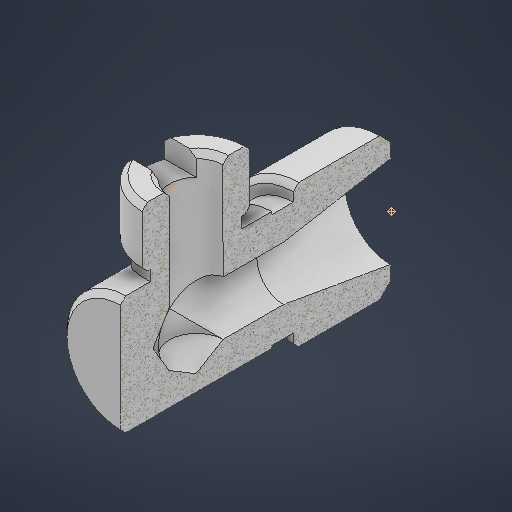
# Autodesk Inventor part: b5
Saved by Autodesk Inventor 2025.4 (Build 294407000, 407)
## iProperties
Created: 2026-05-15
Part Number: b5
Material: Generic
Document SubType Name: Modeling
Designer: VuQuan
Density: 1 g/cm^3
Appearance: Default
Author: VuQuan
Autodesk Inventor part; units mm, degrees
ref_plane "YZ Plane" through (0, 0, 0) normal (1, 0, 0) x (0, 1, 0)
ref_plane "XY Plane" through (0, 0, 0) normal (0, 0, 1) x (1, 0, 0)
sketch "Sketch1" plane through (0, 0, 0) normal (0, 0, 1) x (1, 0, 0)
  circle A0 centre (0, 0) radius 6.58
  circle A1 centre (0, 0) radius 5.5
  circle A2 centre (0, 0) radius 5.25
  dimension "d0" = 13.16
  dimension "d1" = 11
  dimension "d2" = 10.5
  constraints: 3 centre point, 3 coincident
  measures "d0" diameter of A0
  measures "d1" diameter of A1
  measures "d2" diameter of A2
extrude "Extrusion1" add sketch "Sketch1" along normal blind 9 contours A0 | A1 | A2
extrude "Extrusion2" add sketch "Sketch1" along normal blind 2 from surface at 9 contours A2
extrude "Extrusion3" add sketch "Sketch1" along normal blind 14 from surface at 11 contours A1 | A2
sketch "Sketch7" plane through (0, 0, 0) normal (1, 0, 0) x (0, 1, 0)
  line L0 (0, 0) -> (0, 9.9247)
  line L1 (0, 9.9247) -> (2.5, 9.9247)
  line L2 (2.5, 9.9247) -> (4.25, 0)
  line L3 (4.25, 0) -> (0, 0)
  dimension "d71" = 8.5
  dimension "d72" = 10
  dimension "d73" = 2.5
  constraints: 8 end point, 1 horizontal, 1 perpendicular, 1 vertical
  measures "d71" diameter of L2.end L0
  measures "d72" angle of L0 L2
  measures "d73" distance of L0.end L1.end
revolve "Revolution2" cut sketch "Sketch7" angle 360 about axis through (0, 0, 0) along (0, 0, 1)
chamfer "Chamfer2" distance 0.5 angle 45 2 edges at (-6.58, 0, 9) (-5.5, 0, 25)
ref_plane "Work Plane1" through (0, 12, 0) normal (0, 1, 0) x (-1, 0, 0)
sketch "Sketch2" plane through (0, 12, 0) normal (0, 1, 0) x (-1, 0, 0)
  circle A0 centre (0, 18) radius 5
  circle A1 centre (0, 18) radius 2.5
  circle A2 centre (0, 18) radius 4.25
  point P0 (0, 0)
  point P1 (0, 20.5)
  dimension "d17" = 5
  dimension "d16" = 10
  dimension "d18" = 8.5
  constraints: 3 vertical alignment, 2 centre point, 2 coincident, 2 other
  measures "d16" diameter of A0
  measures "d18" diameter of A2
extrude "Extrusion4" add sketch "Sketch2" against normal blind 5.5 contours A0 | A1 | A2
extrude "Extrusion5" add sketch "Sketch2" against normal up to surface from surface at -5.5 contours A1 | A2 round surface about axis through (0, 0, 0) along (0, 0, 1) radius 5.5 far side no
ref_plane "Work Plane2" through (0, -2.5, 0) normal (0, 1, 0) x (-1, 0, 0)
sketch "Sketch6" plane through (0, 12, 18) normal (0, 1, 0) x (1, 0, 0)
  circle A0 centre (0, 0) radius 5 projected
  point P0 (0, 18)
  constraints: 1 coincident
hole "Hole4" at (0, 12, 18) direction (0, -1, 0) diameter 5 depth 14.5 tip angle 118
ref_plane "Work Plane3" through (0, 12, 20.5) normal (0, 0, 1) x (1, 0, 0)
hole "Hole3" at (0, 0, 0) direction (0, 0, 1) diameter 5 depth 20.5 tip angle 118
chamfer "Chamfer5" distance 0.5 angle 45 3 edges at (5, 12, 18) (0, 12, 15.5) (5, 6.5, 18)
chamfer "Chamfer6" distance 1 angle 45 1 edges at (-6.58, 0, 0)
sketch "Sketch8" plane through (0, 0, 0) normal (1, 0, 0) x (0, 1, 0)
  line L0 (12, 15) -> (12, 21) projected
  line L1 (12, 19.75) -> (10, 19.75)
  line L2 (6.5, 13.5) -> (6.5, 22.5) projected
  line L3 (10, 19.75) -> (10, 16.25)
  line L4 (10, 16.25) -> (12, 16.25)
  point P0 (0, 0)
  point P1 (10, 18)
  point P2 (12, 18)
  dimension "d75" = 2
  dimension "d76" = 3.5
  constraints: 6 end point, 2 midpoint, 2 perpendicular, 2 point on line, 1 horizontal alignment, 1 parallel
  measures "d75" distance of L1.start L1.end
  measures "d76" distance between parallel lines of L1 L4
extrude "Extrusion6" cut sketch "Sketch8" along normal through all both and the other way through all
body "Solid1"
